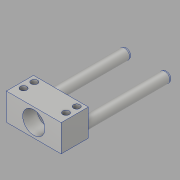
# Autodesk Inventor part: PocketNC_Vise_part1
Saved by Autodesk Inventor 2017 (Build 210142000, 142)
## iProperties
Created: 2018-06-05
Part Number: PocketNC_Vise_part1
Material: Aluminum 6061
Document SubType Name: Modeling
Designer: Jarrett
Density: 2.7 g/cm^3
Appearance: Aluminum - Flat
Author: Jarrett
Autodesk Inventor part; units mm, degrees
ref_plane "YZ Plane" through (0, 0, 0) normal (1, 0, 0) x (0, 1, 0)
ref_plane "XZ Plane" through (0, 0, 0) normal (0, 1, 0) x (-1, 0, 0)
ref_plane "XY Plane" through (0, 0, 0) normal (0, 0, 1) x (1, 0, 0)
sketch "Sketch1" plane through (0, 0, 0) normal (0, 1, 0) x (-1, 0, 0)
  line L0 (12.71, 0) -> (12.71, 12.6)
  line L1 (12.71, 12.6) -> (-12.71, 12.6)
  line L2 (-12.71, 12.6) -> (-12.71, 0)
  line L3 (-12.71, 0) -> (12.71, 0)
  point P0 (0, 0)
  dimension "d0" = 12.71
  dimension "d1" = 12.6
  dimension "d2" = 25.42
  constraints: 8 end point, 2 horizontal, 1 perpendicular
  measures "d0" distance of point (0, 0) L0.start
  measures "d1" distance of L0.start L0.end
  measures "d2" distance of L0.end L1.end
extrude "Extrusion1" add sketch "Sketch1" along normal mid plane 12.56
sketch "Sketch2" plane through (-12.71, 6.28, 12.6) normal (0, 0, 1) x (1, 0, 0)
  circle A0 centre (12.71, -6.28) radius 3.7
  dimension "d5" = 7.4
  constraints: 1 centre point, 1 coincident
  measures "d5" diameter of A0
extrude "Extrusion2" cut sketch "Sketch2" against normal blind 17.3225
sketch "Sketch3" plane through (-12.71, 6.28, 12.6) normal (0, 0, 1) x (1, 0, 0)
  circle A0 centre (12.71, -6.28) radius 5.15
  dimension "d8" = 10.3
  constraints: 1 centre point, 1 coincident
  measures "d8" diameter of A0
extrude "Extrusion3" cut sketch "Sketch3" against normal blind 6.5
sketch "Sketch4" plane through (0, 6.28, 0) normal (0, 1, 0) x (1, 0, 0)
  line L0 (0, 0) -> (-9.85, 0) construction
  line L1 (-9.85, 0) -> (-9.85, -2.5) construction
  circle A0 centre (-9.85, -2.5) radius 1.5
  line L2 (-9.85, -2.5) -> (-9.85, -7.5) construction
  circle A1 centre (-9.85, -7.5) radius 1.5
  circle A2 centre (9.85, -2.5) radius 1.5
  circle A3 centre (9.85, -7.5) radius 1.5
  dimension "d11" = 9.85
  dimension "d12" = 2.5
  dimension "d13" = 3
  dimension "d14" = 5
  dimension "d15" = 3
  constraints: 6 end point, 4 centre point, 2 coincident, 1 perpendicular, 1 vertical
  measures "d11" distance of L0.start L0.end
  measures "d12" distance of L0.end L1.end
  measures "d13" diameter of A0
  measures "d14" distance of L2.start L2.end
  measures "d15" diameter of A1
extrude "Extrusion4" cut sketch "Sketch4" against normal blind 8.2
chamfer "Chamfer1" distance 0.25 angle 45 4 edges at (-11.35, -1.92, 7.5) (-11.35, -1.92, 2.5) (8.35, -1.92, 2.5) (8.35, -1.92, 7.5)
sketch "Sketch5" plane through (12.71, 6.28, 0) normal (0, 0, -1) x (-1, 0, 0)
  line L0 (1, -12.56) -> (1, -9.185) construction
  line L1 (1, -9.185) -> (3.375, -9.185) construction
  circle A0 centre (3.375, -9.185) radius 2.375
  circle A1 centre (12.71, -6.28) radius 3.7 projected
  line L2 (12.71, -12.56) -> (12.71, -6.28) construction
  circle A2 centre (22.045, -9.185) radius 2.375
  point P0 (0, -12.56)
  dimension "d21" = 1
  dimension "d22" = 3.375
  dimension "d23" = 2.375
  constraints: 6 end point, 1 centre point, 1 coincident, 1 horizontal alignment, 1 perpendicular, 1 symmetric about line, 1 vertical, 3 other
  measures "d21" distance of point (0, -12.56) L0.start
  measures "d22" distance of L0.start L0.end
  measures "d23" distance of L0.end L1.end
extrude "Extrusion5" add sketch "Sketch5" along normal blind 39.6 contours A0 | A2
chamfer "Chamfer2" distance 0.25 angle 70 1 edges at (11.71, -2.905, -39.6) measured on face at (9.5733, -3.5643, -39.6)
chamfer "Chamfer3" distance 0.25 angle 70 1 edges at (-6.96, -2.905, -39.6) measured on face at (-9.9756, -2.2535, -39.6)
body "Solid1"
